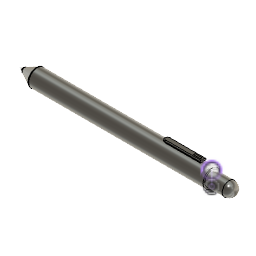
Pen (Autodesk Fusion 360 design; units mm, degrees)
part number: 2026-02-11-19-16-52-477
Autodesk Fusion 360 part; units mm, degrees
sketch "Sketch1" plane through (0, 0, 0) normal (1, 0, 0) x (0, 1, 0)
  circle A0 centre (0, 0) radius 5
  dimension "d1" = 10
  constraint coincident A0.centre origin
  measures "d1" diameter of A0
extrude "Extrude1" add sketch "Sketch1" along normal blind 100 thin wall 1 inside makes body 1
sketch "Sketch2" plane through (0, 0, 0) normal (0, 1, 0) x (1, 0, 0)
  line L0 (0, 0) -> (-10, 0) construction
  line L1 (0, -5) -> (0, 0)
  line L2 (-10, 0) -> (0, -5) construction
  line L3 (0, 0) -> (-7.1399, 0) construction
  line L4 (-7.1399, 0) -> (-7.1399, -1.43) construction
  line L5 (-7.1399, -1.43) -> (0, -1.43) construction
  line L6 (0, -1.43) -> (0, 0) construction
  line L7 (-7.1399, 0) -> (-7.1399, -1.43)
  line L8 (-7.1399, -1.43) -> (0, -5)
  line L9 (0, 0) -> (0, -5)
  line L10 (-7.1399, 0) -> (0, 0)
  dimension "d5" = 10
  constraint coincident L0.start L1.end
  constraint horizontal L0
  constraint perpendicular L0 L1
  constraint horizontal L3
  constraint vertical L4
  constraint horizontal L5
  constraint vertical L6
  constraint coincident L2 L4.end
  measures "d5" distance of L0.start L0.end
revolve "Revolve1" add sketch "Sketch2" angle 360 about axis through (0, 0, 0) along (-1, 0, 0) bodies 1
sketch "Sketch3" plane through (0, 0, 0) normal (0, 1, 0) x (1, 0, 0)
  line L0 (-7.1399, 1.43) -> (-7.1399, -1.43) construction
  line L1 (-7.1399, -1.43) -> (-7.1399, 1.43) construction
  line L2 (-7.1399, -1.43) -> (-7.1399, -1.1) construction
  line L3 (-7.1399, 0) -> (-9.2, 0) construction
  line L4 (-9.2, 0) -> (-9.8542, 0) construction
  line L5 (-9.8542, 0) -> (-7.6568, -1.1)
  line L6 (-7.6568, -1.1) -> (-7.1399, -1.1)
  line L7 (-9.8, 0) -> (-7.1399, 0)
  line L8 (-7.1399, -1.1) -> (-7.1399, 0)
  line L9 (-9.8, 0) -> (-9.8542, 0)
  point P0 (-7.1399, -1.43)
  constraint coincident P0 L0.end
  constraint coincident L0.start L1.end
  constraint coincident L0 L2.end
  constraint midpoint L0 L3.start
  constraint perpendicular L0 L3
  constraint perpendicular L0 L4
  constraint perpendicular L1 L6
  constraint coincident L4 L7.start
revolve "Revolve2" add sketch "Sketch3" angle 360 about axis through (-7.1399, 0, 0) along (-1, 0, 0) bodies 1
fillet "Fillet1" radius 1 1 edges at (0, -4.6616, -1.8081) on bodies 1
sketch "Sketch4" plane through (0, 0, 0) normal (0, 1, 0) x (1, 0, 0)
  line L0 (100, 4) -> (100, -4)
  line L1 (100, 4) -> (100, -4) construction
  constraint coincident L0.start L1.start
  constraint parallel L0 L1
sketch "Sketch5" plane through (100, 0, 0) normal (1, 0, 0) x (0, 1, 0)
  circle A0 centre (0, 0) radius 4
  circle A1 centre (0, 0) radius 5
  circle A2 centre (0, 0) radius 4
  constraint coincident A0.centre A1.centre
extrude "Extrude2" add sketch "Sketch5" along normal blind 10 separate body contours A0 A2 makes body 2
extrude "Extrude3" add 1 faces at (110, -0.7053, 0.7808) along direction (1, 0, 0) blind 4 on bodies 2 bodies 2
fillet "Fillet2" radius 4 1 faces at (114, -0.7053, 0.7808) on bodies 2
sketch "Sketch6" plane through (0, 0, 0) normal (0, 0, 1) x (1, 0, 0)
  line L0 (100, 0) -> (91.8792, 0)
  line L1 (89.8792, 0.5) -> (93.8792, 0.5)
  line L2 (93.8792, 0.5) -> (93.8792, -0.5)
  line L3 (93.8792, -0.5) -> (89.8792, -0.5)
  line L4 (89.8792, -0.5) -> (89.8792, 0.5)
  line L5 (89.8792, 0.5) -> (93.8792, -0.5) construction
  line L6 (93.8792, 0.5) -> (89.8792, -0.5) construction
  point P0 (91.8792, 0)
  dimension "d16" = 4
  dimension "d17" = 1
  constraint horizontal L0
  constraint horizontal L1
  constraint perpendicular L1 L2
  constraint parallel L1 L3
  constraint parallel L2 L4
  constraint coincident L5 P0
  constraint coincident L6 P0
  constraint coincident P0 L0.end
  measures "d16" distance of L2.end L3.end
  measures "d17" distance of L1.end L2.end
extrude "Extrude4" add sketch "Sketch6" along normal blind 7 bodies 1
sketch "Sketch7" plane through (0, 0, 7) normal (0, 0, 1) x (-1, 0, 0)
  line L0 (-89.8792, 0.5) -> (-93.8792, 0.5)
  line L1 (-93.8792, 0.5) -> (-93.8792, -0.5)
  line L2 (-93.8792, -0.5) -> (-89.8792, -0.5)
  line L3 (-89.8792, -0.5) -> (-89.8792, 0.5)
  line L4 (-93.8792, -0.5) -> (-95.0792, -0.5) construction
  line L5 (-95.0792, -0.5) -> (-95.0792, -1.7) construction
  line L6 (-95.0792, -1.7) -> (-93.8792, -1.7) construction
  line L7 (-93.8792, -1.7) -> (-93.8792, -0.5) construction
  line L8 (-95.0792, -1.7) -> (-73.0792, -1.7)
  line L9 (-73.0792, -1.7) -> (-73.0792, 1.7)
  line L10 (-73.0792, 1.7) -> (-95.0792, 1.7)
  line L11 (-95.0792, 1.7) -> (-95.0792, -1.7)
  dimension "d20" = 1.2
  dimension "d21" = 1.2
  dimension "d22" = 22
  dimension "d23" = 3.4
  constraint horizontal L4
  constraint vertical L5
  constraint horizontal L6
  constraint vertical L7
  constraint coincident L1.end L2.start
  constraint horizontal L8
  constraint vertical L9
  constraint horizontal L10
  constraint vertical L11
  measures "d20" distance of L1.end L4.end
  measures "d21" distance of L1.end L6.end
  measures "d22" distance of L5.end L8.end
  measures "d23" distance of L5.end L10.end
extrude "Extrude5" add sketch "Sketch7" along normal blind 1 separate body makes body 3
fillet "Fillet3" radius 0.5 3 edges at (84.0792, 1.7, 8) (84.0792, -1.7, 8) (73.0792, 0, 8) on bodies 3
fillet "Fillet4" radius 1.7 4 edges at (73.2257, 1.5536, 7.8536) (73.0792, 1.7, 7.25) (73.2257, -1.5536, 7.8536) (73.0792, -1.7, 7.25) on bodies 3
move_body "Move1" bodies 3 to x (1, 0, 0) y (0, 1, 0) z (0, 0, 1) at (0, 0, -1)
